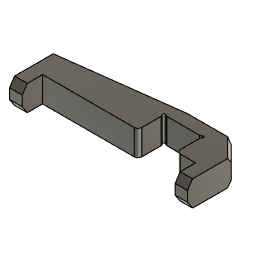
Z Linear Rail Jig v2 (Autodesk Fusion 360 design; units mm, degrees)
Autodesk Fusion 360 part; units mm, degrees
sketch "Sketch1" plane through (0, 0, 0) normal (0, 0, 1) x (1, 0, 0)
  line L0 (0, 0) -> (0, 8)
  line L1 (0, 8) -> (37.55, 8)
  line L2 (37.55, 8) -> (37.55, 18.2)
  line L3 (37.55, 18.2) -> (52.65, 18.2)
  line L4 (52.65, 18.2) -> (52.65, 8)
  line L5 (52.65, 8) -> (60.15, 8)
  line L6 (60.15, 8) -> (60.15, 0)
  line L7 (60.15, 0) -> (65, 0)
  line L8 (65, 0) -> (65, 23.2)
  line L9 (65, 23.2) -> (-5, 23.2)
  line L10 (-5, 23.2) -> (-5, 0)
  line L11 (-5, 0) -> (0, 0)
  dimension "d4" = 10.2
  dimension "d5" = 15.1
  dimension "d6" = 5
  dimension "d7" = 5
  dimension "d8" = 8
  dimension "d26" = 70
  dimension "d27" = 60.15
  dimension "d28" = 7.5
  constraint coincident L0.start L11.end
  constraint vertical L0
  constraint perpendicular L0 L1
  constraint perpendicular L1 L2
  constraint perpendicular L2 L3
  constraint perpendicular L3 L4
  constraint perpendicular L4 L5
  constraint collinear L1 L5
  constraint perpendicular L5 L6
  constraint perpendicular L6 L7
  constraint perpendicular L7 L8
  constraint perpendicular L6 L9
  constraint perpendicular L9 L10
  constraint perpendicular L0 L11
  constraint collinear L7 L11
  measures "d4" distance of L1.end L2.end
  measures "d5" distance of L2.end L3.end
  measures "d6" distance of L0 L10
  measures "d7" distance of L3 L9
  measures "d8" distance of L1 L11
  measures "d26" distance of L8 L10
  measures "d27" distance of L0 L6
  measures "d28" distance of L4.end L5.end
extrude "Extrude1" add sketch "Sketch1" along normal blind 10
chamfer "Chamfer1" distance 6 angle 45 1 edges at (65, 23.2, 5)
chamfer "Chamfer1" distance 39 distance2 5 1 edges at (-5, 23.2, 5) measured on face at (41.6667, 23.2, 3.3333)
fillet "Fillet1" radius 1.5 2 edges at (37.55, 8, 5) (52.65, 8, 5)
sketch "Sketch2" plane through (0, 0, 10) normal (0, 0, 1) x (-1, 0, 0)
  arc A0 (-52.65, -9.5) -> (-54.15, -8) centre (-54.15, -9.5) ccw
  line L0 (-54.15, -8) -> (-60.15, -8)
  line L1 (-60.15, -8) -> (-60.15, 0)
  line L2 (-60.15, 0) -> (-65, 0)
  line L3 (-65, 0) -> (-65, -17.2)
  line L4 (-65, -17.2) -> (-59, -23.2)
  line L5 (-59, -23.2) -> (-34, -23.2)
  line L6 (-34, -23.2) -> (5, -18.2)
  line L7 (5, -18.2) -> (5, 0)
  line L8 (5, 0) -> (0, 0)
  line L9 (0, 0) -> (0, -8)
  line L10 (0, -8) -> (-36.05, -8)
  arc A1 (-36.05, -8) -> (-37.55, -9.5) centre (-36.05, -9.5) ccw
  line L11 (-37.55, -9.5) -> (-37.55, -18.2)
  line L12 (-37.55, -18.2) -> (-52.65, -18.2)
  line L13 (-52.65, -18.2) -> (-52.65, -9.5)
  circle A2 centre (-37.55, -18.2) radius 0.5
  circle A3 centre (-52.65, -18.2) radius 0.5
  dimension "d16" = 1
  constraint coincident L11.end L12.start
  constraint coincident L12.end L13.start
  constraint equal A2 A3
  measures "d16" diameter of A3
extrude "Extrude2" cut sketch "Sketch2" against normal through all contours L12 L13 A3 | L11 L12 A2 picked at (-52.6418, -18.5323) picked at (-37.8815, -18.2248)
fillet "Fillet2" radius 1 4 edges at (37.55, 17.7, 5) (38.05, 18.2, 5) (52.15, 18.2, 5) (52.65, 17.7, 5)
chamfer "Chamfer2" distance 2 distance2 1 4 edges at (14.5, 20.7, 10) (14.5, 20.7, 0) (62, 20.2, 10) (62, 20.2, 0) measured on face at (21, 21.5333, 3.3333) measured on face at (21, 21.5333, 3.3333) measured on face at (61, 21.2, 6.6667) measured on face at (61, 21.2, 6.6667)
chamfer "Chamfer3" distance 2 distance2 3 2 edges at (62.575, 0, 10) (-2.5, 0, 10) measured on face at (10.6882, 14.5041, 10) measured on face at (10.6882, 14.5041, 10)
chamfer "Chamfer3" distance 3 distance2 2 2 edges at (62.575, 0, 0) (-2.5, 0, 0) measured on face at (61.7667, 0, 3.3333) measured on face at (-3.3333, 0, 3.3333)
